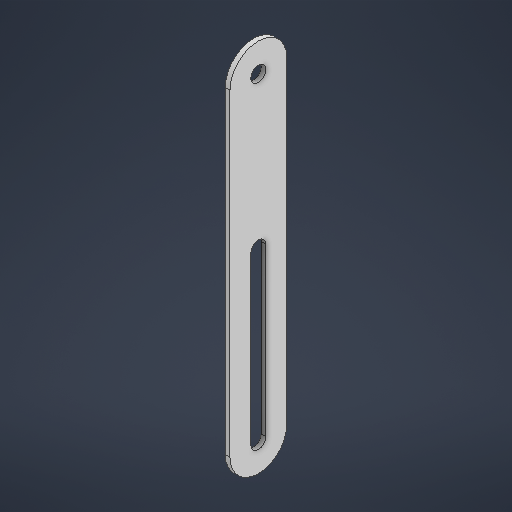
# Autodesk Inventor part: hgsupport
Saved by Autodesk Inventor 2025.2 (Build 292293000, 293)
## iProperties
Created: 2025-04-18
Part Number: hgsupport
Material: Generic
Document SubType Name: Modeling
Designer: roejo
Density: 1 g/cm^3
Appearance: Default
Author: roejo
Autodesk Inventor part; units mm, degrees
ref_plane "YZ Plane" through (0, 0, 0) normal (1, 0, 0) x (0, 1, 0)
ref_plane "XZ Plane" through (0, 0, 0) normal (0, 1, 0) x (-1, 0, 0)
ref_plane "XY Plane" through (0, 0, 0) normal (0, 0, 1) x (1, 0, 0)
sketch "Sketch1" plane through (0, 0, 0) normal (1, 0, 0) x (0, 1, 0)
  circle A0 centre (0, 0) radius 2.54
  arc A1 (0, -9.525) -> (0, 9.525) centre (0, 0) ccw
  line L0 (0, 9.525) -> (-106.68, 9.525)
  line L1 (-106.68, -9.525) -> (0, -9.525)
  arc A2 (-50.8, -2.54) -> (-50.8, 2.54) centre (-50.8, 0) ccw
  line L2 (-50.8, 2.54) -> (-106.68, 2.54)
  line L3 (-106.68, -2.54) -> (-50.8, -2.54)
  line L4 (-109.22, 0) -> (-106.68, 0)
  arc A3 (-106.68, 2.54) -> (-106.68, -2.54) centre (-106.68, 0) ccw
  arc A4 (-106.68, 9.525) -> (-106.68, -9.525) centre (-106.68, 0) ccw
  point P0 (-111.76, 0)
  dimension "d0" = 5.08
  dimension "d12" = 5.08
  dimension "d13" = 2.54
  dimension "d14" = 5.08
  dimension "d15" = 19.05
  constraints: 10 end point, 8 point on circle, 5 centre point, 4 coincident, 3 horizontal, 2 tangent, 1 parallel, 1 point on line
  measures "d0" diameter of A0
  measures "d12" diameter of A2
  measures "d13" distance of L4.start L4.end
  measures "d14" diameter of A3
  measures "d15" diameter of A4
extrude "Extrusion1" add sketch "Sketch1" along normal blind 1.5875
body "Solid1"
